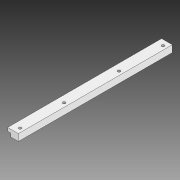
# Autodesk Inventor part: 1324_Clamp Rail_V1
Saved by Autodesk Inventor 2020 (Build 240168000, 168)
## iProperties
Created: 2019-10-02
Part Number: 1324_Clamp Rail_V1
Material: Acetal Resin, White
Document SubType Name: Modeling
Designer: MPI
Density: 1.425 g/cm^3
Appearance: Smooth - White
Author: MPI
Autodesk Inventor part; units mm, degrees
ref_plane "YZ Plane" through (0, 0, 0) normal (1, 0, 0) x (0, 1, 0)
ref_plane "XZ Plane" through (0, 0, 0) normal (0, 1, 0) x (-1, 0, 0)
ref_plane "XY Plane" through (0, 0, 0) normal (0, 0, 1) x (1, 0, 0)
sketch "Sketch1" plane through (0, 0, 0) normal (0, 0, 1) x (1, 0, 0)
  line L0 (14, 12.3) -> (14, 0)
  line L1 (14, 0) -> (0, 0)
  line L2 (0, 0) -> (0, 6.3)
  line L3 (-5.5, 12.3) -> (14, 12.3)
  line L4 (0, 6.3) -> (-5.5, 6.3)
  line L5 (-5.5, 6.3) -> (-5.5, 12.3)
  dimension "d1" = 6.3
  dimension "d2" = 6
  dimension "d4" = 14
  dimension "d5" = 5.5
  constraints: 12 end point, 2 parallel, 1 coincident, 1 horizontal
  measures "d1" distance from line of point (0, 0) L4
  measures "d2" distance of L4.end L3.start
  measures "d4" distance of L0.end L1.end
  measures "d5" distance of L2.end L4.end
extrude "Extrusion1" add sketch "Sketch1" along normal blind 280
sketch "Sketch2" plane through (-5.5, 12.3, 0) normal (0, 1, 0) x (1, 0, 0)
  circle A0 centre (12.5, -270) radius 2.5
  circle A1 centre (12.5, -10) radius 2.5
  circle A2 centre (12.5, -190) radius 2.5
  line L0 (19.5, -280) -> (0, -280) projected
  line L1 (19.5, 0) -> (19.5, -280) projected
  line L2 (19.5, 0) -> (0, 0) projected
  circle A3 centre (12.5, -90) radius 2.5
  point P0 (5.5, 0)
  dimension "d8" = 5
  dimension "d9" = 10
  dimension "d10" = 7
  dimension "d11" = 10
  dimension "d12" = 7
  dimension "d13" = 7
  dimension "d14" = 90
  dimension "d15" = 5
  dimension "d16" = 90
  dimension "d17" = 7
  constraints: 4 centre point, 2 equal radius
  measures "d8" diameter of A0
  measures "d9" distance from line of L0 A0.centre
  measures "d10" distance from line of L1 A0.centre
  measures "d11" distance from line of L2 A1.centre
  measures "d12" distance from line of L1 A1.centre
  measures "d13" distance from line of L1 A2.centre
  measures "d14" distance from line of A2.centre L0
  measures "d15" diameter of A3
  measures "d16" distance from line of A3.centre L2
  measures "d17" distance from line of L1 A3.centre
extrude "Extrusion2" cut sketch "Sketch2" against normal through all
fillet "Fillet1" radius 1 1 edges at (0, 6.3, 140)
body "Solid1"
